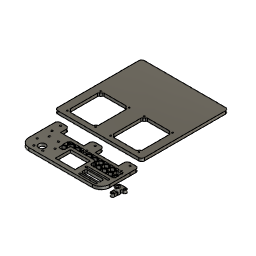
scocca v1.2 (Autodesk Fusion 360 design; units mm, degrees)
Autodesk Fusion 360 part; units mm, degrees
sketch "Schizzo1" plane through (0, 0, 0) normal (0, 0, 1) x (1, 0, 0)
  circle A0 centre (36.25, 84.4234) radius 1.5
  circle A1 centre (28.5, 71) radius 1.5
  circle A2 centre (36.25, 57.5766) radius 1.5
  circle A3 centre (59.5, 71) radius 1.5
  circle A4 centre (51.75, 57.5766) radius 1.5
  circle A5 centre (51.75, 84.4234) radius 1.5
  circle A6 centre (44, 64) radius 6
  line L0 (19.9998, 100) -> (19.9998, 65)
  line L1 (34.9998, 50) -> (145, 50)
  line L2 (160, 100) -> (160, 65)
  line L3 (108, 57) -> (74, 57)
  line L4 (74, 57) -> (74, 83)
  line L5 (74, 83) -> (108, 83)
  line L6 (108, 83) -> (108, 57)
  arc A7 (19.9998, 65) -> (34.9998, 50) centre (34.9998, 65) ccw
  arc A8 (145, 50) -> (160, 65) centre (145, 65) ccw
  line L7 (146, 59) -> (119, 59)
  line L8 (117, 61) -> (117, 65)
  line L9 (119, 67) -> (146, 67)
  line L10 (148, 65) -> (148, 61)
  arc A9 (117, 61) -> (119, 59) centre (119, 61) ccw
  arc A10 (119, 67) -> (117, 65) centre (119, 65) ccw
  arc A11 (148, 65) -> (146, 67) centre (146, 65) ccw
  arc A12 (146, 59) -> (148, 61) centre (146, 61) ccw
  line L11 (113.5, 72.5) -> (151.5, 72.5)
  line L12 (151.5, 69.5) -> (113.5, 69.5)
  line L13 (112, 71) -> (112, 71)
  line L14 (118.5, 53.5) -> (146.5, 53.5)
  line L15 (148, 55) -> (148, 55)
  line L16 (146.5, 56.5) -> (118.5, 56.5)
  line L17 (117, 55) -> (117, 55)
  arc A13 (112, 71) -> (113.5, 69.5) centre (113.5, 71) ccw
  arc A14 (113.5, 72.5) -> (112, 71) centre (113.5, 71) ccw
  arc A15 (148, 55) -> (146.5, 56.5) centre (146.5, 55) ccw
  arc A16 (146.5, 53.5) -> (148, 55) centre (146.5, 55) ccw
  arc A17 (117, 55) -> (118.5, 53.5) centre (118.5, 55) ccw
  arc A18 (118.5, 56.5) -> (117, 55) centre (118.5, 55) ccw
  line L18 (153, 71) -> (153, 71)
  arc A19 (153, 71) -> (151.5, 72.5) centre (151.5, 71) ccw
  arc A20 (151.5, 69.5) -> (153, 71) centre (151.5, 71) ccw
  circle A21 centre (175, 63) radius 2
  circle A22 centre (175, 55) radius 1.5
  circle A23 centre (170, 71) radius 1.5
  circle A24 centre (180, 71) radius 1.5
  line L19 (170, 68) -> (170, 68)
  line L20 (170, 74) -> (180, 74)
  line L21 (180, 68) -> (180, 68)
  arc A25 (170, 74) -> (170, 68) centre (170, 71) ccw
  arc A26 (180, 68) -> (180, 74) centre (180, 71) ccw
  arc A27 (172, 55) -> (178, 55) centre (175, 55) ccw
  arc A28 (172, 66) -> (170, 68) centre (170, 66) ccw
  arc A29 (180, 68) -> (178, 66) centre (180, 66) ccw
  line L22 (155, 91.6603) -> (155, 92)
  line L23 (60, 92) -> (60, 88)
  line L24 (155, 80.5) -> (155, 84.3397)
  line L25 (66, 76) -> (63, 76)
  line L26 (60, 83.0001) -> (60, 88)
  line L27 (87.7434, 91.6972) -> (85.6698, 90.5)
  line L28 (85.6698, 90.5) -> (85.6698, 88)
  line L29 (94.33, 88) -> (94.33, 90.5)
  line L30 (94.33, 90.5) -> (92.2564, 91.6972)
  line L31 (84.33, 88) -> (84.33, 90.5)
  line L32 (84.33, 90.5) -> (79.9999, 93)
  line L33 (79.9999, 93) -> (75.6698, 90.5)
  line L34 (75.6698, 90.5) -> (75.6698, 88)
  line L35 (65.6698, 85.5) -> (69, 83.5773)
  line L36 (74.33, 88) -> (74.33, 90.5)
  line L37 (74.33, 90.5) -> (69.9999, 93)
  line L38 (69.9999, 93) -> (65.6698, 90.5)
  line L39 (65.6698, 90.5) -> (65.6698, 85.5)
  line L40 (59.9999, 83) -> (64.33, 85.5)
  line L41 (64.33, 85.5) -> (64.33, 90.5)
  line L42 (64.33, 90.5) -> (60.1436, 92.917)
  line L43 (104.33, 88) -> (104.33, 90.5)
  line L44 (104.33, 90.5) -> (99.9999, 93)
  line L45 (99.9999, 93) -> (95.6698, 90.5)
  line L46 (95.6698, 90.5) -> (95.6698, 88)
  line L47 (113, 84.7321) -> (114.33, 85.5)
  line L48 (114.33, 85.5) -> (114.33, 90.5)
  line L49 (114.33, 90.5) -> (109.9999, 93)
  line L50 (109.9999, 93) -> (105.6698, 90.5)
  line L51 (105.6698, 90.5) -> (105.6698, 88)
  line L52 (115.6698, 85.5) -> (119.9999, 83)
  line L53 (119.9999, 83) -> (124.33, 85.5)
  line L54 (124.33, 85.5) -> (124.33, 90.5)
  line L55 (124.33, 90.5) -> (119.9999, 93)
  line L56 (119.9999, 93) -> (115.6698, 90.5)
  line L57 (115.6698, 90.5) -> (115.6698, 85.5)
  line L58 (125.6698, 85.5) -> (129.9999, 83)
  line L59 (129.9999, 83) -> (134.33, 85.5)
  line L60 (134.33, 85.5) -> (134.33, 90.5)
  line L61 (134.33, 90.5) -> (129.9999, 93)
  line L62 (129.9999, 93) -> (125.6698, 90.5)
  line L63 (125.6698, 90.5) -> (125.6698, 85.5)
  line L64 (135.6698, 85.5) -> (139.9999, 83)
  line L65 (139.9999, 83) -> (144.33, 85.5)
  line L66 (144.33, 85.5) -> (144.33, 90.5)
  line L67 (144.33, 90.5) -> (139.9999, 93)
  line L68 (139.9999, 93) -> (135.6698, 90.5)
  line L69 (135.6698, 90.5) -> (135.6698, 85.5)
  line L70 (145.6698, 85.5) -> (149.9999, 83)
  line L71 (149.9999, 83) -> (154.33, 85.5)
  line L72 (154.33, 85.5) -> (154.33, 90.5)
  line L73 (154.33, 90.5) -> (152.2564, 91.6972)
  line L74 (147.7435, 91.6973) -> (145.6698, 90.5)
  line L75 (145.6698, 90.5) -> (145.6698, 85.5)
  line L76 (119.33, 77.5) -> (119.3301, 81.8396)
  line L77 (119.3301, 81.8396) -> (115, 84.3397)
  line L78 (115, 84.3397) -> (113, 83.1851)
  line L79 (129.33, 77.5) -> (129.3301, 81.8396)
  line L80 (129.3301, 81.8396) -> (125, 84.3397)
  line L81 (125, 84.3397) -> (120.6698, 81.8399)
  line L82 (120.6698, 81.8399) -> (120.6697, 77.5)
  line L83 (139.33, 77.5) -> (139.3301, 81.8396)
  line L84 (139.3301, 81.8396) -> (135, 84.3397)
  line L85 (135, 84.3397) -> (130.6698, 81.8399)
  line L86 (130.6698, 81.8399) -> (130.6697, 77.5)
  line L87 (149.33, 77.5) -> (149.3301, 81.8396)
  line L88 (149.3301, 81.8396) -> (145, 84.3397)
  line L89 (145, 84.3397) -> (140.6698, 81.8399)
  line L90 (140.6698, 81.8399) -> (140.6697, 77.5)
  line L91 (155, 84.3397) -> (150.6698, 81.8399)
  line L92 (150.6698, 81.8399) -> (150.6697, 77.5)
  line L93 (69, 82.0302) -> (65, 84.3397)
  line L94 (65, 84.3397) -> (60.6698, 81.8399)
  line L95 (60.6698, 81.8399) -> (60.6697, 77.1107)
  line L96 (95, 91.6603) -> (99.3301, 94.1604)
  line L97 (99.3301, 94.1604) -> (99.33, 95)
  line L98 (100.6698, 95) -> (100.6698, 94.1601)
  line L99 (100.6698, 94.1601) -> (105, 91.6603)
  line L100 (105, 91.6603) -> (109.3301, 94.1604)
  line L101 (109.3301, 94.1604) -> (109.33, 95)
  line L102 (110.6698, 95) -> (110.6698, 94.1601)
  line L103 (110.6698, 94.1601) -> (115, 91.6603)
  line L104 (115, 91.6603) -> (119.3301, 94.1604)
  line L105 (119.3301, 94.1604) -> (119.33, 95)
  line L106 (120.6698, 95) -> (120.6698, 94.1601)
  line L107 (120.6698, 94.1601) -> (125, 91.6603)
  line L108 (125, 91.6603) -> (129.3301, 94.1604)
  line L109 (129.3301, 94.1604) -> (129.33, 95)
  line L110 (130.6698, 95) -> (130.6698, 94.1601)
  line L111 (130.6698, 94.1601) -> (135, 91.6603)
  line L112 (135, 91.6603) -> (139.3301, 94.1604)
  line L113 (139.3301, 94.1604) -> (139.33, 95)
  line L114 (140.6698, 95) -> (140.6698, 94.1601)
  line L115 (140.6698, 94.1601) -> (145, 91.6603)
  line L116 (153.2512, 92.6699) -> (155, 91.6603)
  line L117 (80.6698, 95) -> (80.6698, 94.1601)
  line L118 (80.6698, 94.1601) -> (85, 91.6603)
  line L119 (70.6698, 95) -> (70.6698, 94.1601)
  line L120 (70.6698, 94.1601) -> (75, 91.6603)
  line L121 (75, 91.6603) -> (79.3301, 94.1604)
  line L122 (79.3301, 94.1604) -> (79.33, 95)
  line L123 (60.8276, 94.069) -> (65, 91.6603)
  line L124 (65, 91.6603) -> (69.3301, 94.1604)
  line L125 (69.3301, 94.1604) -> (69.33, 95)
  arc A30 (60.6697, 77.1107) -> (63, 76) centre (63, 79) ccw
  arc A31 (66, 76) -> (69, 79) centre (66, 79) ccw
  arc A32 (72, 88) -> (69, 85) centre (72, 85) ccw
  arc A33 (113, 80.5) -> (116, 77.5) centre (116, 80.5) ccw
  arc A34 (113, 85) -> (110, 88) centre (110, 85) ccw
  arc A35 (152, 77.5) -> (155, 80.5) centre (152, 80.5) ccw
  arc A36 (155, 92) -> (153.9367, 94.2911) centre (152, 92) ccw
  line L126 (72, 88) -> (74.33, 88)
  line L127 (69, 85) -> (69, 83.5773)
  line L128 (69, 82.0302) -> (69, 79)
  arc A37 (63, 95) -> (60.8276, 94.069) centre (63, 92) ccw
  arc A38 (60.1436, 92.917) -> (60, 92) centre (63, 92) ccw
  line L129 (69.33, 95) -> (63, 95)
  line L130 (79.33, 95) -> (70.6698, 95)
  line L131 (75.6698, 88) -> (84.33, 88)
  line L132 (113, 85) -> (113, 84.7321)
  line L133 (113, 83.1851) -> (113, 80.5)
  line L134 (105.6698, 88) -> (110, 88)
  line L135 (85.6698, 88) -> (94.33, 88)
  line L136 (95.6698, 88) -> (104.33, 88)
  line L137 (99.33, 95) -> (93.9999, 95)
  line L138 (109.33, 95) -> (100.6698, 95)
  line L139 (119.33, 95) -> (110.6698, 95)
  line L140 (116, 77.5) -> (119.33, 77.5)
  line L141 (120.6697, 77.5) -> (129.33, 77.5)
  line L142 (130.6697, 77.5) -> (139.33, 77.5)
  line L143 (140.6697, 77.5) -> (149.33, 77.5)
  line L144 (150.6697, 77.5) -> (152, 77.5)
  line L145 (139.33, 95) -> (130.6698, 95)
  line L146 (129.33, 95) -> (120.6698, 95)
  line L147 (172, 55) -> (172, 59.6834)
  arc A39 (178.3333, 60.7889) -> (178.2, 65.4) centre (175, 63) ccw
  arc A40 (171.8, 65.4) -> (171.6667, 60.7889) centre (175, 63) ccw
  line L148 (178, 55) -> (178, 59.6834)
  arc A41 (172, 59.6834) -> (171.6667, 60.7889) centre (170, 59.6834) ccw
  arc A42 (178.3333, 60.7889) -> (178, 59.6834) centre (180, 59.6834) ccw
  arc A43 (171.8, 65.4) -> (172, 66) centre (171, 66) ccw
  arc A44 (178, 66) -> (178.2, 65.4) centre (179, 66) ccw
  line L149 (39.9998, 100) -> (39.9998, 110)
  line L150 (34.9998, 115) -> (24.9998, 115)
  line L151 (19.9998, 110) -> (19.9998, 100)
  line L152 (79.9999, 100) -> (79.9999, 110)
  line L153 (84.9999, 115) -> (89.9999, 115)
  line L154 (99.9999, 100) -> (99.9999, 110)
  line L155 (94.9999, 115) -> (89.9999, 115)
  line L156 (145, 115) -> (155, 115)
  line L157 (160, 110) -> (160, 100)
  line L158 (140, 100) -> (140, 110)
  line L159 (140, 100) -> (99.9999, 100)
  line L160 (79.9999, 100) -> (39.9998, 100)
  arc A45 (24.9998, 115) -> (19.9998, 110) centre (24.9998, 110) ccw
  arc A46 (39.9998, 110) -> (34.9998, 115) centre (34.9998, 110) ccw
  arc A47 (84.9999, 115) -> (79.9999, 110) centre (84.9999, 110) ccw
  arc A48 (99.9999, 110) -> (94.9999, 115) centre (94.9999, 110) ccw
  arc A49 (145, 115) -> (140, 110) centre (145, 110) ccw
  arc A50 (160, 110) -> (155, 115) centre (155, 110) ccw
  line L161 (29.9998, 115) -> (29.9998, 110)
  circle A51 centre (29.9998, 110) radius 1.5
  circle A52 centre (89.9999, 110) radius 1.5
  circle A53 centre (150, 110) radius 1.5
  circle A54 centre (30, 95) radius 1.5
  circle A55 centre (89.9999, 95) radius 1.5
  circle A56 centre (150, 95) radius 1.5
  line L162 (85.9999, 95) -> (80.6698, 95)
  line L163 (85, 91.6603) -> (86.7486, 92.6699)
  arc A57 (85.9999, 95) -> (86.7486, 92.6699) centre (89.9999, 95) ccw
  arc A58 (87.7434, 91.6972) -> (92.2564, 91.6972) centre (89.9999, 95) ccw
  arc A59 (93.2511, 92.6699) -> (93.9999, 95) centre (89.9999, 95) ccw
  line L164 (93.2511, 92.6699) -> (95, 91.6603)
  arc A60 (147.7435, 91.6973) -> (152.2564, 91.6972) centre (150, 95) ccw
  arc A61 (153.2512, 92.6699) -> (153.9367, 94.2911) centre (150, 95) ccw
  arc A62 (146, 95) -> (146.7487, 92.6699) centre (150, 95) ccw
  line L165 (146, 95) -> (140.6698, 95)
  line L166 (145, 91.6603) -> (146.7487, 92.6699)
  line L167 (150, 135) -> (150, 275)
  line L168 (145, 280) -> (5, 280)
  line L169 (0, 275) -> (0, 135)
  circle A63 centre (88, 138.5) radius 1.25
  line L170 (137, 144.1569) -> (137, 190.8431)
  circle A64 centre (88, 196.5) radius 1.25
  circle A65 centre (137, 196.5) radius 1.25
  circle A66 centre (137, 138.5) radius 1.25
  arc A67 (89.3333, 192.7288) -> (91.7712, 195.1667) centre (88, 196.5) ccw
  arc A68 (91.7712, 139.8333) -> (89.3333, 142.2712) centre (88, 138.5) ccw
  line L171 (88, 190.8431) -> (88, 144.1569)
  line L172 (93.6569, 138.5) -> (131.3431, 138.5)
  arc A69 (135.6667, 142.2712) -> (133.2288, 139.8333) centre (137, 138.5) ccw
  line L173 (131.3431, 196.5) -> (93.6569, 196.5)
  arc A70 (133.2288, 195.1667) -> (135.6667, 192.7288) centre (137, 196.5) ccw
  arc A71 (93.6569, 196.5) -> (91.7712, 195.1667) centre (93.6569, 194.5) ccw
  arc A72 (89.3333, 192.7288) -> (88, 190.8431) centre (90, 190.8431) ccw
  arc A73 (88, 144.1569) -> (89.3333, 142.2712) centre (90, 144.1569) ccw
  arc A74 (91.7712, 139.8333) -> (93.6569, 138.5) centre (93.6569, 140.5) ccw
  arc A75 (131.3431, 138.5) -> (133.2288, 139.8333) centre (131.3431, 140.5) ccw
  arc A76 (135.6667, 142.2712) -> (137, 144.1569) centre (135, 144.1569) ccw
  arc A77 (137, 190.8431) -> (135.6667, 192.7288) centre (135, 190.8431) ccw
  arc A78 (133.2288, 195.1667) -> (131.3431, 196.5) centre (131.3431, 194.5) ccw
  arc A79 (60.6667, 142.2712) -> (58.2288, 139.8333) centre (62, 138.5) ccw
  line L174 (18.6569, 196.5) -> (56.3431, 196.5)
  line L175 (56.3431, 138.5) -> (18.6569, 138.5)
  arc A80 (14.3333, 192.7288) -> (13, 190.8431) centre (15, 190.8431) ccw
  circle A81 centre (13, 138.5) radius 1.25
  arc A82 (18.6569, 196.5) -> (16.7712, 195.1667) centre (18.6569, 194.5) ccw
  arc A83 (60.6667, 142.2712) -> (62, 144.1569) centre (60, 144.1569) ccw
  arc A84 (13, 144.1569) -> (14.3333, 142.2712) centre (15, 144.1569) ccw
  arc A85 (56.3431, 138.5) -> (58.2288, 139.8333) centre (56.3431, 140.5) ccw
  arc A86 (58.2288, 195.1667) -> (56.3431, 196.5) centre (56.3431, 194.5) ccw
  arc A87 (16.7712, 139.8333) -> (14.3333, 142.2712) centre (13, 138.5) ccw
  arc A88 (14.3333, 192.7288) -> (16.7712, 195.1667) centre (13, 196.5) ccw
  arc A89 (62, 190.8431) -> (60.6667, 192.7288) centre (60, 190.8431) ccw
  circle A90 centre (62, 138.5) radius 1.25
  arc A91 (16.7712, 139.8333) -> (18.6569, 138.5) centre (18.6569, 140.5) ccw
  circle A92 centre (62, 196.5) radius 1.25
  line L176 (62, 190.8431) -> (62, 144.1569)
  circle A93 centre (13, 196.5) radius 1.25
  line L177 (13, 144.1569) -> (13, 190.8431)
  arc A94 (58.2288, 195.1667) -> (60.6667, 192.7288) centre (62, 196.5) ccw
  line L178 (5, 130) -> (145, 130)
  arc A95 (5, 280) -> (0, 275) centre (5, 275) ccw
  arc A96 (150, 275) -> (145, 280) centre (145, 275) ccw
  arc A97 (145, 130) -> (150, 135) centre (145, 135) ccw
  arc A98 (0, 135) -> (5, 130) centre (5, 135) ccw
  point P0 (89.9999, 88)
  point P1 (94.9999, 79.3397)
  point P2 (94.9999, 96.6603)
  dimension "d27" = 3
  dimension "d28" = 3
  dimension "d29" = 12
  dimension "d32" = 15
  dimension "d38" = 1.5
  dimension "d40" = 1.5
  dimension "d41" = 1.5
  dimension "d43" = 4
  dimension "d44" = 3
  dimension "d52" = 2
  dimension "d53" = 2
  dimension "d65" = 3
  dimension "d67" = 2
  dimension "d68" = 1
  dimension "d73" = 5
  dimension "d74" = 3
  dimension "d75" = 3
  dimension "d76" = 3
  dimension "d77" = 3
  dimension "d90" = 2.5
  dimension "d93" = 2.5
  dimension "d94" = 2.5
  dimension "d95" = 2.5
  dimension "d100" = 8
  dimension "d101" = 2
  dimension "d102" = 5
  constraint perpendicular L0 L159
  constraint perpendicular L0 L1
  constraint horizontal L3
  constraint vertical L4
  constraint horizontal L5
  constraint vertical L6
  constraint tangent L0 A7
  constraint tangent L1 A7
  constraint tangent L1 A8
  constraint tangent L2 A8
  constraint equal A7 A8
  constraint horizontal L7
  constraint vertical L8
  constraint horizontal L9
  constraint tangent L7 A9
  constraint tangent L8 A9
  constraint tangent L8 A10
  constraint tangent L9 A10
  constraint equal A9 A10
  constraint tangent L9 A11
  constraint equal A9 A11
  constraint horizontal L11
  constraint horizontal L12
  constraint horizontal L14
  constraint horizontal L16
  constraint tangent L12 A13
  constraint tangent L11 A14
  constraint equal A13 A14
  constraint tangent L16 A15
  constraint tangent L14 A16
  constraint equal A15 A16
  constraint tangent L14 A17
  constraint equal A15 A17
  constraint tangent L16 A18
  constraint equal A15 A18
  constraint tangent L11 A19
  constraint tangent L12 A20
  constraint equal A19 A20
  constraint concentric A23 A25
  constraint tangent A27 L147
  constraint vertical L147
  constraint tangent L20 A26
  constraint tangent A27 L148
  constraint vertical L148
  constraint tangent A28 L147
  constraint tangent A29 L148
  constraint horizontal L126
  constraint vertical L22
  constraint vertical L23
  constraint vertical L132
  constraint horizontal L140
  constraint vertical L24
  constraint vertical L127
  constraint horizontal L25
  constraint vertical L26
  constraint tangent L23 A37
  constraint tangent L25 A30
  constraint tangent L26 A30
  constraint equal A30 A37
  constraint tangent A31 L127
  constraint tangent L25 A31
  constraint equal A31 A37
  constraint tangent A32 L127
  constraint tangent A32 L126
  constraint equal A32 A37
  constraint tangent A33 L132
  constraint tangent A33 L140
  constraint equal A33 A37
  constraint tangent A34 L132
  constraint tangent A34 L126
  constraint equal A34 A37
  constraint tangent A35 L140
  constraint tangent L24 A35
  constraint equal A35 A37
  constraint tangent L22 A36
  constraint equal A36 A37
  constraint coincident L34.end L126
  constraint collinear L126 L131
  constraint collinear L127 L128
  constraint coincident L40 L26.start
  constraint coincident L42.end A37
  constraint concentric A37 A38
  constraint collinear L131 L135
  constraint coincident L78.end L132
  constraint collinear L132 L133
  constraint coincident L51.end L135
  constraint collinear L134 L135
  constraint coincident L46.end L135
  constraint collinear L135 L136
  constraint collinear L140 L141
  constraint coincident L86.end L141
  constraint collinear L141 L142
  constraint collinear L142 L143
  constraint coincident L92.end L143
  constraint collinear L143 L144
  constraint collinear L145 L146
  constraint concentric A21 A39
  constraint concentric A39 A40
  constraint tangent L147 A41
  constraint tangent A40 A41
  constraint tangent A39 A42
  constraint tangent L148 A42
  constraint equal A41 A42
  constraint tangent A28 A43
  constraint tangent A40 A43
  constraint tangent A29 A44
  constraint tangent A39 A44
  constraint equal A43 A44
  constraint vertical L149
  constraint horizontal L150
  constraint vertical L151
  constraint vertical L152
  constraint horizontal L153
  constraint collinear L159 L160
  constraint tangent L150 A45
  constraint tangent L151 A45
  constraint tangent L149 A46
  constraint tangent L150 A46
  constraint equal A45 A46
  constraint tangent L153 A47
  constraint tangent L152 A47
  constraint equal A45 A47
  constraint tangent L154 A48
  constraint tangent L155 A48
  constraint equal A45 A48
  constraint tangent L156 A49
  constraint tangent L158 A49
  constraint equal A45 A49
  constraint tangent L156 A50
  constraint tangent L157 A50
  constraint equal A45 A50
  constraint midpoint L150 L161.start
  constraint perpendicular L150 L161
  constraint coincident L161.end A51.centre
  constraint concentric A55 A58
  constraint concentric A56 A60
  constraint coincident L162.start A58
  constraint concentric A57 A58
  constraint concentric A58 A59
  constraint concentric A60 A61
  constraint concentric A61 A62
  constraint vertical L167
  constraint horizontal L168
  constraint vertical L169
  constraint horizontal L172
  constraint vertical L170
  constraint concentric A63 A68
  constraint concentric A66 A69
  constraint concentric A64 A67
  constraint concentric A65 A70
  constraint tangent A67 A71
  constraint tangent L173 A71
  constraint tangent L171 A72
  constraint tangent A67 A72
  constraint equal A71 A72
  constraint tangent A68 A73
  constraint tangent L171 A73
  constraint equal A71 A73
  constraint tangent A68 A74
  constraint tangent L172 A74
  constraint equal A71 A74
  constraint tangent L172 A75
  constraint tangent A69 A75
  constraint equal A71 A75
  constraint tangent L170 A76
  constraint tangent A69 A76
  constraint equal A71 A76
  constraint tangent A70 A77
  constraint tangent L170 A77
  constraint equal A71 A77
  constraint tangent L173 A78
  constraint tangent A70 A78
  constraint equal A71 A78
  constraint perpendicular L167 L178
  constraint tangent L168 A95
  constraint tangent L169 A95
  constraint tangent L167 A96
  constraint tangent L168 A96
  constraint equal A95 A96
  constraint tangent L167 A97
  constraint tangent L178 A97
  constraint equal A95 A97
  constraint tangent L169 A98
  constraint tangent L178 A98
  constraint equal A95 A98
  measures "d27" diameter of A0
  measures "d28" diameter of A1
  measures "d29" diameter of A6
  measures "d32" radius of A7
  measures "d38" radius of A13
  measures "d40" radius of A15
  measures "d41" radius of A19
  measures "d43" diameter of A21
  measures "d44" diameter of A22
  measures "d52" radius of A28
  measures "d53" radius of A29
  measures "d65" radius of A37
  measures "d67" radius of A41
  measures "d68" radius of A43
  measures "d73" radius of A45
  measures "d74" diameter of A51
  measures "d75" diameter of A52
  measures "d76" diameter of A53
  measures "d77" diameter of A54
  measures "d90" diameter of A63
  measures "d93" diameter of A64
  measures "d94" diameter of A65
  measures "d95" diameter of A66
  measures "d100" diameter of A70
  measures "d101" radius of A71
  measures "d102" radius of A95
extrude "Extrude1" add sketch "Schizzo1" along normal blind 5 makes body 1 at (70.769, 252.5706, 0) makes body 2 at (62.4134, 61.4906, 0) makes body 3 at (173.8942, 69.399, 0)
sketch "Sketch2" plane through (0, 0, 5) normal (0, 0, 1) x (-1, 0, 0)
  circle A0 centre (-170, -71) radius 1.5
  circle A1 centre (-180, -71) radius 1.5
  circle A2 centre (-175, -55) radius 1.5
  circle A3 centre (-175, -63) radius 2
  arc A4 (-180, -68) -> (-180, -74) centre (-180, -71) ccw
  line L0 (-180, -74) -> (-170, -74)
  arc A5 (-170, -74) -> (-170, -68) centre (-170, -71) ccw
  arc A6 (-172, -66) -> (-170, -68) centre (-170, -66) ccw
  arc A7 (-171.8, -65.4) -> (-172, -66) centre (-171, -66) ccw
  arc A8 (-171.8, -65.4) -> (-171.6667, -60.7889) centre (-175, -63) ccw
  arc A9 (-172, -59.6834) -> (-171.6667, -60.7889) centre (-170, -59.6834) ccw
  line L1 (-172, -59.6834) -> (-172, -55)
  arc A10 (-172, -55) -> (-178, -55) centre (-175, -55) ccw
  line L2 (-178, -55) -> (-178, -59.6834)
  arc A11 (-178.3333, -60.7889) -> (-178, -59.6834) centre (-180, -59.6834) ccw
  arc A12 (-178.3333, -60.7889) -> (-178.2, -65.4) centre (-175, -63) ccw
  arc A13 (-178, -66) -> (-178.2, -65.4) centre (-179, -66) ccw
  arc A14 (-180, -68) -> (-178, -66) centre (-180, -66) ccw
  circle A15 centre (-175, -63) radius 2
  circle A16 centre (-175, -63) radius 4
  constraint concentric A3 A15
  constraint concentric A15 A16
extrude "Extrude2" add sketch "Sketch2" along normal blind 5 contours A8 A12 A16 bodies 3
